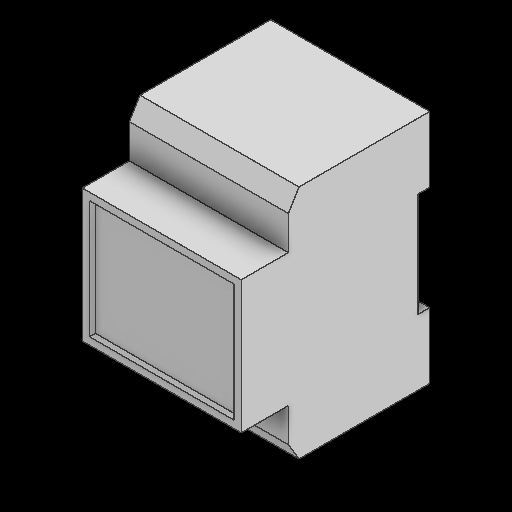
# Autodesk Inventor part: EnergyMeter
Saved by Autodesk Inventor 2025.2 (Build 292293000, 293)
## iProperties
Created: 2026-05-14
Part Number: EnergyMeter
Material: Generic
Document SubType Name: Modeling
Designer: valer
Density: 1 g/cm^3
Appearance: Default
Author: valer
Autodesk Inventor part; units mm, degrees
ref_plane "YZ Plane" through (0, 0, 0) normal (1, 0, 0) x (0, 1, 0)
ref_plane "XZ Plane" through (0, 0, 0) normal (0, 1, 0) x (-1, 0, 0)
ref_plane "XY Plane" through (0, 0, 0) normal (0, 0, 1) x (1, 0, 0)
sketch "Base" plane through (0, 0, 0) normal (0, 0, 1) x (1, 0, 0)
  line L0 (-27, -40) -> (27, -40)
  line L1 (27, -40) -> (27, 40)
  line L2 (27, 40) -> (-27, 40)
  line L3 (-27, 40) -> (-27, -40)
  line L4 (-27, -40) -> (27, 40) construction
  line L5 (27, -40) -> (-27, 40) construction
  point P0 (0, 0)
  dimension "d0" = 80
  dimension "d1" = 54
  constraints: 12 end point, 2 midpoint, 2 parallel, 1 horizontal, 1 perpendicular
  measures "d0" distance of L2.end L0.start
  measures "d1" distance of L0.start L0.end
extrude "BaseFeature" add sketch "Base" along normal blind 48
sketch "DINRail" plane through (-27, -40, 0) normal (-1, 0, 0) x (0, 0, 1)
  line L0 (0, 80) -> (0, 0) construction
  line L1 (0, 0) -> (48, 0) construction
  line L2 (48, 80) -> (48, 0) construction
  line L3 (0, 80) -> (48, 80) construction
  line L4 (0, 57.7) -> (4, 57.7)
  line L5 (4, 57.7) -> (4, 22.3)
  line L6 (4, 22.3) -> (0, 22.3)
  line L7 (0, 22.3) -> (0, 57.7)
  line L8 (0, 57.7) -> (4, 22.3) construction
  line L9 (4, 57.7) -> (0, 22.3) construction
  line L10 (0, -16) -> (0, 96) projected
  line L11 (-9.6, 40) -> (57.6, 40) construction
  line L12 (0, 80) -> (0, 0) projected
  point P0 (2, 40)
  point P1 (0, -16)
  point P2 (0, 96)
  dimension "d4" = 4
  dimension "d5" = 35.4
  constraints: 12 end point, 2 midpoint, 2 parallel, 1 horizontal, 1 perpendicular, 1 point on line, 1 vertical, 2 other
  measures "d4" distance of L4.start L4.end
  measures "d5" distance of L6.end L4.start
extrude "DinRailFeature" cut sketch "DINRail" against normal through all
sketch "Chamfers" plane through (-27, -40, 48) normal (-1, 0, 0) x (0, 0, 1)
  line L0 (-44, 22.3) -> (-48, 22.3) construction
  line L1 (-48, 22.3) -> (-48, 0) construction
  line L2 (-48, 0) -> (0, 0) projected
  line L3 (0, 80) -> (0, 0) projected
  line L4 (-48, 80) -> (0, 80) projected
  line L5 (-48, 80) -> (-48, 57.7) construction
  line L6 (-48, 57.7) -> (-44, 57.7) construction
  line L7 (-44, 57.7) -> (-44, 22.3) construction
  line L8 (-3.6, 80) -> (0, 74)
  line L9 (-57.6, 40) -> (9.6, 40) construction
  line L10 (-3.6, 0) -> (0, 6)
  point P0 (-48, 40)
  point P1 (0, 6)
  point P2 (-3.6, 0)
  dimension "d8" = 6
  dimension "d9" = 3.6
  constraints: 4 end point, 2 point on line, 2 symmetric about line
  measures "d8" distance of L8.end L3.start
  measures "d9" distance of L3.start L8.start
extrude "ChamfersFeature" cut sketch "Chamfers" against normal through all
sketch "Screen" plane through (0, 0, 48) normal (0, 0, 1) x (1, 0, 0)
  line L0 (27, -34) -> (27, 34) projected
  line L1 (-27, 22.5) -> (27, 22.5)
  line L2 (27, 22.5) -> (27, -22.5)
  line L3 (27, -22.5) -> (-27, -22.5)
  line L4 (-27, -22.5) -> (-27, 22.5)
  line L5 (-27, 22.5) -> (27, -22.5) construction
  line L6 (27, 22.5) -> (-27, -22.5) construction
  point P0 (0, 0)
  dimension "d12" = 45
  constraints: 12 end point, 2 midpoint, 2 parallel, 1 horizontal, 1 perpendicular, 1 point on line
  measures "d12" distance between parallel lines of L3 L1
extrude "ScreenFeature" add sketch "Screen" along normal blind 16
sketch "ScreenBezel" plane through (0, 0, 64) normal (0, 0, 1) x (1, 0, 0)
  line L0 (-24.5, -20) -> (24.5, -20)
  line L1 (24.5, -20) -> (24.5, 20)
  line L2 (24.5, 20) -> (-24.5, 20)
  line L3 (-24.5, 20) -> (-24.5, -20)
  line L4 (-24.5, -20) -> (24.5, 20) construction
  line L5 (24.5, -20) -> (-24.5, 20) construction
  line L6 (27, 22.5) -> (-27, 22.5) projected
  line L7 (27, -22.5) -> (27, 22.5) projected
  point P0 (0, 0)
  dimension "d15" = 2.5
  dimension "d16" = 2.5
  constraints: 12 end point, 2 midpoint, 2 parallel, 1 horizontal, 1 perpendicular
  measures "d15" distance between parallel lines of L6 L2
  measures "d16" distance between parallel lines of L7 L1
extrude "ScreenBezelFeature" cut sketch "ScreenBezel" against normal blind 1
chamfer "ScreenChamferFeature" distance 1 angle 45 4 edges at (-24.5, 0, 63) (0, 20, 63) (24.5, 0, 63) (0, -20, 63)
sketch "SupplyTerminals" plane through (0, 0, 48) normal (0, 0, 1) x (1, 0, 0)
  line L0 (-27, -40) -> (27, -40) projected
  line L1 (-27, -34) -> (27, -34) projected
  line L2 (-22, -40) -> (-16, -40)
  line L3 (-16, -40) -> (-16, -34)
  line L4 (-16, -34) -> (-22, -34)
  line L5 (-22, -34) -> (-22, -40)
  circle A0 centre (-19, -34) radius 3
  line L6 (-27, -40) -> (-27, -34) projected
  line L7 (27, -22.5) -> (-27, -22.5) projected
  line L8 (-14, -22.5) -> (-14, -40) construction
  line L9 (-6, -40) -> (-12, -40)
  line L10 (-12, -40) -> (-12, -34)
  line L11 (-6, -34) -> (-6, -40)
  circle A1 centre (-9, -34) radius 3
  point P0 (0, 0)
  dimension "d23" = 6
  dimension "d24" = 5
  dimension "d25" = 2
  constraints: 16 end point, 5 symmetric about line, 4 point on line, 2 parallel, 2 perpendicular, 1 horizontal, 1 midpoint, 1 vertical, 6 other
  measures "d23" distance between parallel lines of L3 L5
  measures "d24" distance between parallel lines of L6 L5
  measures "d25" distance between parallel lines of L3 L8
extrude "SupplyTerminalsFeature" cut sketch "SupplyTerminals" against normal up to surface (3.6 mm away) contours L5 A0 L3 L0 | A0 L1 | L1 A0 | L10 A1 L11 L0 | A1 L1 | L1 A1
sketch "TerminalScrews" plane through (-19, -34, 44.4) normal (0, 0, 1) x (1, 0, 0)
  arc A0 (3, 0) -> (-3, 0) centre (0, 0) ccw projected
  arc A1 (13, 0) -> (7, 0) centre (10, 0) ccw projected
  circle A2 centre (0, 0) radius 2.5
  circle A3 centre (10, 0) radius 2.5
  point P0 (19, 34)
  dimension "d28" = 5
  constraints: 2 centre point, 2 coincident, 1 equal radius
  measures "d28" diameter of A2
extrude "TerminalScrewsFeature" cut sketch "TerminalScrews" against normal blind 1
body "Solid1"
